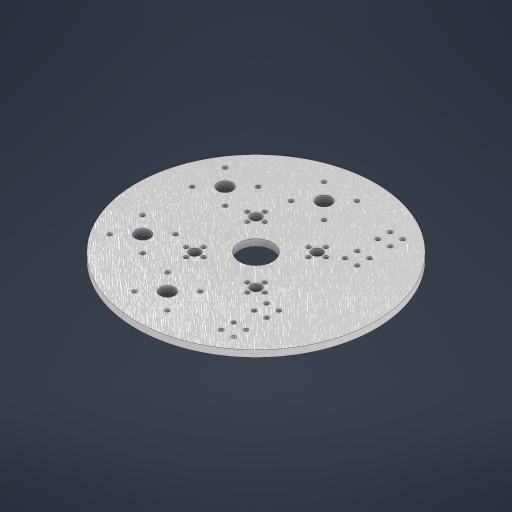
# Autodesk Inventor part: TurnTableTop
Saved by Autodesk Inventor 2024 (Build 280153000, 153)
## iProperties
Created: 2023-10-18
Part Number: TurnTableTop
Material: Generic
Document SubType Name: Modeling
Designer: avsar
Density: 1 g/cm^3
Appearance: Polished Brushed
Author: avsar
Autodesk Inventor part; units mm, degrees
ref_plane "YZ Plane" through (0, 0, 0) normal (1, 0, 0) x (0, 1, 0)
ref_plane "XZ Plane" through (0, 0, 0) normal (0, 1, 0) x (-1, 0, 0)
ref_plane "XY Plane" through (0, 0, 0) normal (0, 0, 1) x (1, 0, 0)
sketch "Sketch1" plane through (0, 0, 0) normal (0, 1, 0) x (-1, 0, 0)
  circle A0 centre (0, 0) radius 116
  dimension "d0" = 232
  constraints: 1 centre point, 1 coincident
  measures "d0" diameter of A0
extrude "Extrusion1" add sketch "Sketch1" along normal mid plane 6.35
sketch "Sketch2" plane through (0, 3.175, 0) normal (0, 1, 0) x (1, 0, 0)
  circle A0 centre (-42, 0) radius 5
  circle A1 centre (-36, 6) radius 2
  circle A2 centre (-48, 6) radius 2
  circle A3 centre (-48, -6) radius 2
  circle A4 centre (-36, -6) radius 2
  circle A5 centre (0, -42) radius 5
  circle A6 centre (-6, -36) radius 2
  circle A7 centre (-6, -48) radius 2
  circle A8 centre (6, -48) radius 2
  circle A9 centre (6, -36) radius 2
  circle A10 centre (42, 0) radius 5
  circle A11 centre (36, -6) radius 2
  circle A12 centre (48, -6) radius 2
  circle A13 centre (48, 6) radius 2
  circle A14 centre (36, 6) radius 2
  circle A15 centre (0, 42) radius 5
  circle A16 centre (6, 36) radius 2
  circle A17 centre (6, 48) radius 2
  circle A18 centre (-6, 48) radius 2
  circle A19 centre (-6, 36) radius 2
  point P0 (0, 0)
  dimension "d3" = 10
  dimension "d4" = 42
  dimension "d5" = 4
  dimension "d6" = 6
  dimension "d7" = 6
  dimension "d10" = 360
  dimension "d14" = 360
  constraints: 20 centre point, 1 horizontal alignment, 50 other
  measures "d3" diameter of A0
  measures "d4" distance of point (0, 0) A0.centre
  measures "d5" diameter of A1
  measures "d6" horizontal distance of A0.centre A1.centre
  measures "d7" horizontal distance of A0.centre A1.centre
extrude "Extrusion2" cut sketch "Sketch2" against normal through all
sketch "Sketch3" plane through (0, 3.175, 0) normal (0, 1, 0) x (1, 0, 0)
  circle A0 centre (0, 0) radius 16
  dimension "d18" = 32
  constraints: 1 centre point, 1 coincident
  measures "d18" diameter of A0
extrude "Extrusion3" cut sketch "Sketch3" against normal through all
move or copy body "Move Body1" bodies to move or copy 1 copy no rotation origin (0, 0, 0) rotation axis (0, 1, 0) rotation angle -45
sketch "Sketch4" plane through (0, 3.175, 0) normal (0, 1, 0) x (1, 0, 0)
  circle A0 centre (0, 0) radius 16 construction
  line L0 (-16, 0) -> (16, 0) construction
  line L1 (0, 16) -> (0, -16) construction
  circle A1 centre (54.2525, -76) radius 2.5 construction
  circle A2 centre (48.2525, -82) radius 2
  circle A3 centre (60.2525, -82) radius 2
  circle A4 centre (60.2525, -70) radius 2
  circle A5 centre (48.2525, -70) radius 2
  line L2 (54.2525, -76) -> (54.2525, -44) construction
  circle A6 centre (54.2525, -44) radius 2.5 construction
  circle A7 centre (48.2525, -50) radius 2
  circle A8 centre (60.2525, -50) radius 2
  circle A9 centre (60.2525, -38) radius 2
  circle A10 centre (48.2525, -38) radius 2
  circle A11 centre (54.2525, 76) radius 2.5 construction
  circle A12 centre (48.2525, 82) radius 2
  circle A13 centre (60.2525, 82) radius 2
  circle A14 centre (60.2525, 70) radius 2
  circle A15 centre (48.2525, 70) radius 2
  line L3 (54.2525, 76) -> (54.2525, 44) construction
  circle A16 centre (54.2525, 44) radius 2.5 construction
  circle A17 centre (48.2525, 50) radius 2
  circle A18 centre (60.2525, 50) radius 2
  circle A19 centre (60.2525, 38) radius 2
  circle A20 centre (48.2525, 38) radius 2
  dimension "d35" = 5
  dimension "d37" = 4
  dimension "d38" = 6
  dimension "d39" = 6
  dimension "d42" = 360
  dimension "d44" = 32
  dimension "d45" = 5
  dimension "d46" = 4
  dimension "d47" = 6
  dimension "d48" = 6
  dimension "d51" = 360
  dimension "d78" = 76
  constraints: 20 centre point, 11 symmetric about line, 8 end point, 4 point on circle, 2 coincident, 2 midpoint, 1 horizontal, 1 perpendicular, 1 vertical, 28 other
  measures "d35" diameter of A1
  measures "d37" diameter of A2
  measures "d38" horizontal distance of L2.start A2.centre
  measures "d39" horizontal distance of L2.start A2.centre
  measures "d44" distance of L2.start L2.end
  measures "d45" diameter of A6
  measures "d46" diameter of A7
  measures "d47" horizontal distance of L2.end A7.centre
  measures "d48" horizontal distance of L2.end A7.centre
  measures "d78" vertical distance of L2.start point (0, 0)
extrude "Extrusion4" cut sketch "Sketch4" against normal through all
sketch "Sketch5" plane through (0, 3.175, 0) normal (0, 1, 0) x (1, 0, 0)
  circle A0 centre (-10, 76) radius 7
  circle A1 centre (-26, 92) radius 2
  circle A2 centre (-26, 60) radius 2
  circle A3 centre (6, 60) radius 2
  circle A4 centre (6, 92) radius 2
  circle A5 centre (0, 0) radius 16 construction
  line L0 (-16, 0) -> (16, 0) construction
  circle A6 centre (-10, -76) radius 7
  circle A7 centre (-26, -92) radius 2
  circle A8 centre (-26, -60) radius 2
  circle A9 centre (6, -60) radius 2
  circle A10 centre (6, -92) radius 2
  line L1 (0, 16) -> (0, -16) construction
  circle A11 centre (-70, 40) radius 7
  circle A12 centre (-54, 56) radius 2
  circle A13 centre (-86, 56) radius 2
  circle A14 centre (-86, 24) radius 2
  circle A15 centre (-54, 24) radius 2
  circle A16 centre (-70, -40) radius 7
  circle A17 centre (-54, -56) radius 2
  circle A18 centre (-86, -56) radius 2
  circle A19 centre (-86, -24) radius 2
  circle A20 centre (-54, -24) radius 2
  dimension "d55" = 14
  dimension "d56" = 10
  dimension "d57" = 76
  dimension "d58" = 4
  dimension "d59" = 16
  dimension "d60" = 16
  dimension "d63" = 360
  dimension "d67" = 14
  dimension "d68" = 4
  dimension "d69" = 16
  dimension "d70" = 16
  dimension "d71" = 40
  dimension "d75" = 360
  dimension "d79" = 70
  constraints: 20 centre point, 10 symmetric about line, 4 end point, 4 point on circle, 2 midpoint, 1 coincident, 1 horizontal, 1 vertical, 28 other
  measures "d55" diameter of A0
  measures "d56" horizontal distance of A0.centre point (0, 0)
  measures "d57" vertical distance of A0.centre point (0, 0)
  measures "d58" diameter of A1
  measures "d59" horizontal distance of A0.centre A1.centre
  measures "d60" horizontal distance of A0.centre A1.centre
  measures "d67" diameter of A11
  measures "d68" diameter of A12
  measures "d69" horizontal distance of A11.centre A12.centre
  measures "d70" horizontal distance of A11.centre A12.centre
  measures "d71" vertical distance of point (0, 0) A11.centre
  measures "d79" horizontal distance of point (0, 0) A11.centre
extrude "Extrusion5" cut sketch "Sketch5" against normal through all
body "Solid1"
